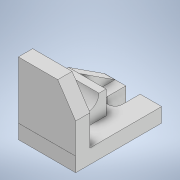
# Autodesk Inventor part: Exercise01
Saved by Autodesk Inventor 2021 (Build 250183000, 183)
## iProperties
Created: 2022-03-17
Part Number: Exercise01
Material: Generic
Document SubType Name: Modeling
Designer: User
Density: 1 g/cm^3
Appearance: Default
Author: User
Autodesk Inventor part; units mm, degrees
ref_plane "YZ Plane" through (0, 0, 0) normal (1, 0, 0) x (0, 1, 0)
ref_plane "XZ Plane" through (0, 0, 0) normal (0, 1, 0) x (-1, 0, 0)
ref_plane "XY Plane" through (0, 0, 0) normal (0, 0, 1) x (1, 0, 0)
sketch "Sketch1" plane through (0, 0, 0) normal (0, 1, 0) x (-1, 0, 0)
  line L0 (37.9585, -11.217) -> (-26.0415, -11.217)
  line L1 (-26.0415, -11.217) -> (-26.0415, -107.217)
  line L2 (-26.0415, -107.217) -> (37.9585, -107.217)
  line L3 (37.9585, -107.217) -> (37.9585, -11.217)
  line L4 (13.9585, -107.217) -> (13.9585, -87.217)
  arc A0 (13.9585, -87.217) -> (-2.0415, -87.217) centre (5.9585, -87.217) ccw
  line L5 (-2.0415, -87.217) -> (-2.0415, -107.217)
  point P0 (0, 0)
  dimension "d0" = 64
  dimension "d1" = 96
  dimension "d2" = 20
  dimension "d3" = 8
  dimension "d4" = 32
  constraints: 12 end point, 2 parallel, 2 perpendicular, 2 point on circle, 2 point on line, 2 tangent, 1 centre point, 1 horizontal
  measures "d0" distance of L2.end L1.end
  measures "d1" distance of L1.end L0.end
  measures "d2" distance of L4.start L4.end
  measures "d3" radius of A0
  measures "d4" distance from line of A0.centre L3
extrude "Extrusion1" add sketch "Sketch1" along normal blind 16 contours L3 L2 L4 A0 L5 L1 L0
sketch "Sketch2" plane through (0, 16, 0) normal (0, 1, 0) x (1, 0, 0)
  line L0 (-37.9585, 11.1917) -> (26.0415, 11.1917)
  line L1 (26.0415, 11.1917) -> (26.0415, 27.1917)
  line L2 (26.0415, 27.1917) -> (-37.9585, 27.1917)
  line L3 (-37.9585, 27.1917) -> (-37.9585, 11.1917)
  line L4 (26.0415, 11.217) -> (26.0415, 107.217) projected
  line L5 (-37.9585, 107.217) -> (-37.9585, 11.217) projected
  point P0 (0, 0)
  dimension "d7" = 16
  constraints: 8 end point, 2 collinear, 2 parallel, 1 horizontal, 1 perpendicular
  measures "d7" distance of L2.end L0.start
extrude "Extrusion2" add sketch "Sketch2" along normal blind 64
chamfer "Chamfer1" distance 20 distance2 30 1 edges at (26.0415, 80, -19.1917) measured on face at (4.7081, 80, -16.525)
sketch "Sketch4" plane through (-37.9585, 0, -107.217) normal (-1, 0, 0) x (0, 0, 1)
  line L0 (80.0253, 15.9344) -> (80.0253, 41.9344)
  line L1 (80.0253, 41.9344) -> (72.0253, 41.9344)
  arc A0 (48.0253, 41.9344) -> (72.0253, 41.9344) centre (60.0253, 41.9344) ccw
  line L2 (48.0253, 41.9344) -> (40.0253, 41.9344)
  line L3 (40.0253, 41.9344) -> (40.0253, 15.9344)
  line L4 (40.0253, 15.9344) -> (80.0253, 15.9344)
  line L5 (80.0253, 16) -> (80.0253, 80) projected
  point P0 (107.217, 0)
  dimension "d19" = 26
  dimension "d20" = 8
  dimension "d21" = 8
  dimension "d22" = 12
  constraints: 10 end point, 3 perpendicular, 2 point on circle, 1 centre point, 1 collinear, 1 horizontal, 1 point on line, 1 vertical
  measures "d19" distance of L0.start L0.end
  measures "d20" distance of L0.end L1.end
  measures "d21" distance of L2.start L2.end
  measures "d22" radius of A0
extrude "Extrusion4" add sketch "Sketch4" against normal blind 42
sketch "Sketch5" plane through (-37.9585, 0, -107.217) normal (-1, 0, 0) x (0, 0, 1)
  line L0 (40.044, 41.902) -> (0.0026, 15.8826)
  line L1 (0.0026, 15.8826) -> (40.044, 15.8826)
  line L2 (40.044, 15.8826) -> (40.044, 41.902)
  point P0 (107.217, 0)
  constraints: 6 end point, 1 horizontal, 1 perpendicular
extrude "Extrusion5" add sketch "Sketch5" against normal blind 12
equation "\"d4\" = 0.5 * d0"
body "Solid1"
